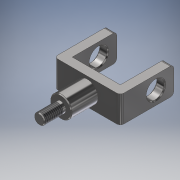
# Autodesk Inventor part: Forcella movimento lama
Saved by Autodesk Inventor 2018 (Build 220112000, 112)
## iProperties
Created: 2020-06-12
Part Number: Forcella movimento lama
Material: Acciaio inossidabile
Document SubType Name: Modeling
Designer: Francesco
Density: 8 g/cm^3
Appearance: Semilucidato
Author: Francesco
Autodesk Inventor part; units mm, degrees
ref_plane "YZ Plane" through (0, 0, 0) normal (1, 0, 0) x (0, 1, 0)
ref_plane "XZ Plane" through (0, 0, 0) normal (0, 1, 0) x (-1, 0, 0)
ref_plane "XY Plane" through (0, 0, 0) normal (0, 0, 1) x (1, 0, 0)
sketch "Schizzo1" plane through (0, 0, 0) normal (0, 0, 1) x (1, 0, 0)
  line L0 (-18.5, 30) -> (-18.5, 0)
  line L1 (-18.5, 0) -> (18.5, 0)
  line L2 (18.5, 0) -> (18.5, 30)
  line L3 (18.5, 30) -> (13.5, 30)
  line L4 (13.5, 30) -> (13.5, 5)
  line L5 (13.5, 5) -> (-13.5, 5)
  line L6 (-13.5, 5) -> (-13.5, 30)
  line L7 (-13.5, 30) -> (-18.5, 30)
  point P0 (0, 0)
  point P1 (0, 5)
  point P2 (0, 0)
  dimension "d0" = 37
  dimension "d1" = 27
  dimension "d2" = 5
  dimension "d3" = 30
  constraints: 16 end point, 7 perpendicular, 2 midpoint, 1 coincident, 1 point on line, 1 vertical, 1 vertical alignment
  measures "d0" distance between parallel lines of L2 L0
  measures "d1" distance between parallel lines of L4 L6
  measures "d2" distance between parallel lines of L1 L5
  measures "d3" distance between parallel lines of L1 L7
extrude "Estrusione1" add sketch "Schizzo1" along normal blind 15
sketch "Schizzo2" plane through (0, 0, 0) normal (1, 0, 0) x (0, 1, 0)
  line L0 (5, 0) -> (30, 0) projected
  line L1 (30, 0) -> (30, 15) projected
  line L2 (5, 15) -> (30, 15) projected
  line L3 (5, 0) -> (5, 15) projected
  circle A0 centre (20, 7.5) radius 5
  point P0 (0, 0)
  point P1 (30, 7.5)
  point P2 (17.5, 0)
  dimension "d6" = 10
  dimension "d23" = 10
  constraints: 2 midpoint, 1 centre point, 1 coincident, 1 horizontal alignment
  measures "d6" diameter of A0
  measures "d23" distance of point (30, 7.5) A0.centre
extrude "Estrusione2" cut sketch "Schizzo2" along normal through all both and the other way through all contours A0
fillet "Raccordo1" radius 2 6 edges at (-16, 30, 15) (-16, 30, 0) (16, 30, 15) (16, 30, 0) (18.5, 0, 7.5) (-18.5, 0, 7.5)
sketch "Schizzo3" plane through (-16.5, 0, 0) normal (0, -1, 0) x (1, 0, 0)
  line L0 (0, 0) -> (0, 15) projected
  line L1 (0, 0) -> (33, 0) projected
  line L2 (33, 15) -> (33, 0) projected
  line L3 (0, 15) -> (33, 15) projected
  circle A0 centre (16.5, 7.5) radius 6
  point P0 (16.5, 0)
  point P1 (33, 7.5)
  point P2 (16.5, 0)
  dimension "d13" = 12
  constraints: 2 midpoint, 1 centre point, 1 coincident, 1 horizontal alignment, 1 vertical alignment
  measures "d13" diameter of A0
extrude "Estrusione3" add sketch "Schizzo3" along normal blind 15 contours A0
sketch "Schizzo4" plane through (0, -15, 7.5) normal (0, -1, 0) x (1, 0, 0)
  circle A0 centre (0, 0) radius 3
  point P0 (0, -7.5)
  dimension "d16" = 6
  constraints: 1 centre point
  measures "d16" diameter of A0
extrude "Estrusione4" add sketch "Schizzo4" along normal blind 12
chamfer "Smusso1" distance 0.5 angle 45 6 edges at (-13.5, 15, 7.5) (13.5, 15, 7.5) (-18.5, 15, 7.5) (18.5, 15, 7.5) (-3, -27, 7.5) (-6, -15, 7.5)
thread "Filettatura2" size "M6x1" class "6g" standard "ANSI Metric M Profile" length 10
